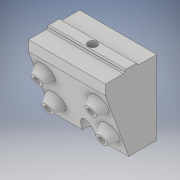
# Autodesk Inventor part: 2020-PiCam2-Angled-Mount
Saved by Autodesk Inventor 2019 (Build 230136000, 136)
## iProperties
Created: 2020-12-31
Part Number: 2020-PiCam2-Angled-Mount
Material: Generic
Document SubType Name: Modeling
Designer: Keith
Density: 1 g/cm^3
Appearance: Default
Author: Keith
## iProperties of the stored document 2020-PiCam2-Angled-Mount_3DPrint.ipt
Created: 2020-12-31
Part Number: 2020-PiCam2-Angled-Mount_3DPrint
Material: Generic
Document SubType Name: Modeling
Designer: Keith
Density: 1 g/cm^3
Appearance: Default
Author: Keith
Autodesk Inventor part; units mm, degrees
ref_plane "YZ Plane" through (0, 0, 0) normal (1, 0, 0) x (0, 1, 0)
ref_plane "XZ Plane" through (0, 0, 0) normal (0, 1, 0) x (-1, 0, 0)
ref_plane "XY Plane" through (0, 0, 0) normal (0, 0, 1) x (1, 0, 0)
sketch "Sketch1" plane through (0, 0, 0) normal (0, 1, 0) x (-1, 0, 0)
  line L0 (0, 0) -> (20, 0)
  line L1 (20, 0) -> (20, -20)
  line L2 (20, -20) -> (0, -20)
  line L3 (0, -20) -> (0, 0)
  dimension "d0" = 20
  dimension "d1" = 20
  constraints: 8 end point, 2 parallel, 1 horizontal, 1 perpendicular
  measures "d0" distance of L1.end L2.end
  measures "d1" distance of L0.end L1.end
extrude "Extrusion1" add sketch "Sketch1" along normal blind 4
sketch "Sketch2" plane through (0, 4, 0) normal (0, 1, 0) x (1, 0, 0)
  line L0 (-20, 0) -> (0, 0) projected
  line L1 (0, 0) -> (0, 20) projected
  line L2 (0, 20) -> (-20, 20) projected
  line L3 (-20, 20) -> (-20, 0) projected
  line L4 (-20, 20) -> (-20, 0) projected
  line L5 (-20, 12.5) -> (0, 12.5)
  line L6 (0, 12.5) -> (0, 7.5)
  line L7 (0, 7.5) -> (-20, 7.5)
  line L8 (-20, 7.5) -> (-20, 12.5)
  dimension "d4" = 7.5
  dimension "d5" = 5
  constraints: 8 end point, 2 parallel, 2 point on line, 1 horizontal, 1 perpendicular
  measures "d4" distance between parallel lines of L0 L7
  measures "d5" distance between parallel lines of L7 L5
extrude "Extrusion2" add sketch "Sketch2" along normal blind 1 contours L3 L5 L1 L7
fillet "Fillet1" radius 0.5 4 edges at (-10, 5, -7.5) (-10, 4, -7.5) (-10, 5, -12.5) (-10, 4, -12.5)
sketch "Sketch3" plane through (-20, 0, -20) normal (-1, 0, 0) x (0, 0, 1)
  arc A0 (8, 5) -> (7.5, 4.5) centre (8, 4.5) ccw projected
  arc A1 (7, 4) -> (7.5, 4.5) centre (7, 4.5) ccw projected
  line L0 (0, 4) -> (7, 4) projected
  line L1 (0, 0) -> (0, 4) projected
  line L2 (20, 0) -> (0, 0) projected
  line L3 (20, 0) -> (20, 4) projected
  line L4 (13, 4) -> (20, 4) projected
  arc A2 (12.5, 4.5) -> (13, 4) centre (13, 4.5) ccw projected
  arc A3 (12.5, 4.5) -> (12, 5) centre (12, 4.5) ccw projected
  line L5 (8, 5) -> (12, 5) projected
  line L6 (20, 0) -> (0, 0) projected
  line L7 (20, 0) -> (39.3501, 0) construction
  line L8 (0, 0) -> (0, -25)
  line L9 (0, -25) -> (10.9007, -25)
  line L10 (20, 0) -> (20, 4) projected
  line L11 (10.9007, -25) -> (20, 0)
  dimension "d10" = 25
  constraints: 8 end point, 2 perpendicular, 1 horizontal
  measures "d10" distance of L1.start L8.end
extrude "Extrusion3" add sketch "Sketch3" against normal up to surface (20 mm away) contours L2 L11 L9 L8
sketch "Sketch5" plane through (-20, 4, -20) normal (-1, 0, 0) x (0, 0, 1)
  arc A0 (8, 1) -> (7.5, 0.5) centre (8, 0.5) ccw projected
  arc A1 (7, 0) -> (7.5, 0.5) centre (7, 0.5) ccw projected
  line L0 (0, 0) -> (7, 0) projected
  line L1 (0, 0) -> (0, -29) projected
  line L2 (0, -29) -> (10.9007, -29) projected
  line L3 (10.9007, -29) -> (20, -4) projected
  line L4 (20, -4) -> (20, 0) projected
  line L5 (13, 0) -> (20, 0) projected
  arc A2 (12.5, 0.5) -> (13, 0) centre (13, 0.5) ccw projected
  arc A3 (12.5, 0.5) -> (12, 1) centre (12, 0.5) ccw projected
  line L6 (8, 1) -> (12, 1) projected
extrude "Extrusion4" add sketch "Sketch5" along normal blind 10
sketch "Sketch6" plane through (-30, 0, 0) normal (0, -0.3420201, 0.9396926) x (1, 0, 0)
  line L0 (30, -26.6044) -> (30, 0) projected
  line L1 (30, 0) -> (0, 0) projected
  line L2 (0, -26.6044) -> (0, 0) projected
  line L3 (30, -26.6044) -> (0, -26.6044) projected
  line L4 (25.5, -18.5466) -> (4.5, -18.5466)
  line L5 (4.5, -18.5466) -> (4.5, -6.0466)
  line L6 (4.5, -6.0466) -> (25.5, -6.0466)
  line L7 (25.5, -6.0466) -> (25.5, -18.5466)
  line L8 (30, -0.0466) -> (0, -0.0466) projected
  dimension "d17" = 21
  dimension "d18" = 12.5
  dimension "d19" = 4.5
  dimension "d22" = 4.5
  dimension "d23" = 6
  constraints: 8 end point, 4 coincident, 2 parallel, 1 horizontal, 1 perpendicular
  measures "d17" distance of L5.end L6.end
  measures "d18" distance of L4.end L5.end
  measures "d19" distance between parallel lines of L2 L5
  measures "d22" distance between parallel lines of L0 L7
  measures "d23" distance between parallel lines of L8 L6
hole "Hole1" at (-4.5, -17.4281, -6.3433) at (-4.5, -5.682, -2.0681) at (-25.5, -5.682, -2.0681) at (-25.5, -17.4281, -6.3433) direction (0, 0.3420201, -0.9396926) diameter 2.4 end through all clearance for "Flat Head Machine Screw" size "M2" standard "Ansi Metric M Profile"
ref_plane "Work Plane1" through (-30, 6.8404, -18.7939) normal (0, -0.3420201, 0.9396926) x (1, 0, 0)
sketch "Sketch8" plane through (-30, 6.8404, -18.7939) normal (0, -0.3420201, 0.9396926) x (1, 0, 0)
  circle A0 centre (4.5, -6.0466) radius 1.2 projected
  circle A1 centre (25.5, -18.5466) radius 1.2 projected
  circle A2 centre (25.5, -6.0466) radius 1.2 projected
  circle A3 centre (4.5, -18.5466) radius 1.2 projected
  line L0 (30, -3.0816) -> (0, -3.0816) projected
  line L1 (30, -3.0816) -> (30, -30.3327) projected
  line L2 (30, -30.3327) -> (0, -30.3327) projected
  line L3 (0, -3.0816) -> (0, -30.3327) projected
  circle A4 centre (4.5, -18.5466) radius 2
  circle A5 centre (4.5, -6.0466) radius 2
  circle A6 centre (25.5, -6.0466) radius 2
  circle A7 centre (25.5, -18.5466) radius 2
  point P0 (30, 0)
  dimension "d32" = 4
  dimension "d33" = 4
  dimension "d34" = 4
  dimension "d35" = 4
  constraints: 4 centre point, 4 coincident
  measures "d32" diameter of A4
  measures "d33" diameter of A5
  measures "d34" diameter of A6
  measures "d35" diameter of A7
extrude "Extrusion5" cut sketch "Sketch8" along normal blind 18 contours A0 | A2 | A4 | A5 | A6 | A7
sketch "Sketch9" plane through (-30, 0, 0) normal (0, -0.3420201, 0.9396926) x (1, 0, 0)
  circle A0 centre (4.5, -6.0466) radius 1.2 projected
  circle A1 centre (25.5, -18.5466) radius 1.2 projected
  circle A2 centre (25.5, -6.0466) radius 1.2 projected
  circle A3 centre (4.5, -18.5466) radius 1.2 projected
  line L0 (30, -26.6044) -> (30, 0) projected
  line L1 (30, 0) -> (0, 0) projected
  line L2 (0, -26.6044) -> (0, 0) projected
  line L3 (30, -26.6044) -> (0, -26.6044) projected
  circle A4 centre (25.5, -18.5466) radius 2.2
  circle A5 centre (4.5, -18.5466) radius 2.2
  circle A6 centre (4.5, -6.0466) radius 2.2
  circle A7 centre (25.5, -6.0466) radius 2.2
  dimension "d38" = 4.4
  dimension "d39" = 4.4
  dimension "d40" = 4.4
  dimension "d41" = 4.4
  constraints: 4 centre point, 4 coincident
  measures "d38" diameter of A4
  measures "d39" diameter of A5
  measures "d40" diameter of A6
  measures "d41" diameter of A7
extrude "Extrusion6" add sketch "Sketch9" along normal blind 3.5 contours A4 | A5 | A6 | A7
chamfer "Chamfer1" distance 1.5 distance2 3.5 1 edges at (-27.7, -17.4281, -6.3433) measured on face at (-28.2, -17.4281, -6.3433)
chamfer "Chamfer2" distance 1.5 distance2 3.5 1 edges at (-27.7, -5.682, -2.0681) measured on face at (-28.2, -5.682, -2.0681)
chamfer "Chamfer3" distance 1.5 distance2 3.5 1 edges at (-6.7, -5.682, -2.0681) measured on face at (-7.2, -5.682, -2.0681)
chamfer "Chamfer4" distance 1.5 distance2 3.5 1 edges at (-6.7, -17.4281, -6.3433) measured on face at (-7.2, -17.4281, -6.3433)
sketch "Sketch10" plane through (0, -25, -20) normal (0, -1, 0) x (1, 0, 0)
  line L0 (0, 8) -> (-30, 8) projected
  line L1 (0, 0) -> (0, 10.9007) projected
  line L2 (0, 10.9007) -> (-30, 10.9007) projected
  line L3 (-30, 0) -> (-30, 10.9007) projected
  line L4 (0, 0) -> (-30, 0) projected
  line L5 (0, 12) -> (-30, 12) projected
  circle A0 centre (-15, 10) radius 2.75
  circle A1 centre (-15, 10) radius 1.7
  point P0 (0, 20)
  dimension "d56" = 2
  dimension "d57" = 15
  dimension "d58" = 5.5
  dimension "d59" = 3.4
  constraints: 2 centre point, 2 coincident
  measures "d56" distance from line of L5 A0.centre
  measures "d57" distance from line of L1 A0.centre
  measures "d58" diameter of A0
  measures "d59" diameter of A1
hole "Hole2" at (-15, -25, -10) direction (0, 1, 0) diameter 3.4 end through all counterbore diameter 6.5 counterbore depth 24 clearance for "Socket Head Cap Screw" size "M3" standard "Ansi Metric M Profile"
body "Solid1"
